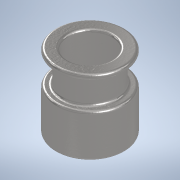
# Autodesk Inventor part: Umlenkrolle
Saved by Autodesk Inventor 2021 (Build 250183000, 183)
## iProperties
Created: 2020-05-16
Part Number: Umlenkrolle
Material: Generisch
Document SubType Name: Modeling
Designer: kaebi
Density: 1 g/cm^3
Appearance: Galvanized
Description: Antriebswelle Zahnriemen (Bestand)
Stock Number: -
Author: kaebi
Autodesk Inventor part; units mm, degrees
ref_plane "YZ Plane" through (0, 0, 0) normal (1, 0, 0) x (0, 1, 0)
ref_plane "XZ Plane" through (0, 0, 0) normal (0, 1, 0) x (-1, 0, 0)
ref_plane "XY Plane" through (0, 0, 0) normal (0, 0, 1) x (1, 0, 0)
sketch "Skizze1" plane through (0, 0, 0) normal (0, 0, 1) x (1, 0, 0)
  line L0 (0, 14) -> (-6.5, 14)
  line L1 (-6.5, 14) -> (-6.5, 13)
  line L2 (-6.5, 13) -> (-5, 13)
  line L3 (-5, 13) -> (-5, 8)
  line L4 (-5, 8) -> (-6.5, 8)
  line L5 (-6.5, 8) -> (-6.5, 0)
  line L6 (-6.5, 0) -> (0, 0)
  line L7 (0, 0) -> (-6.5, 0)
  line L8 (0, 0) -> (0, 14)
  line L9 (0, 13.1706) -> (0, 10.9789)
  dimension "d0" = 8
  dimension "d1" = 5
  dimension "d2" = 1
  dimension "d3" = 10
  dimension "d4" = 13
  constraints: 20 end point, 7 perpendicular, 2 collinear, 2 point on line, 1 horizontal
  measures "d0" distance of L4.end L5.end
  measures "d1" distance of L2.end L3.end
  measures "d2" distance of L0.end L1.end
  measures "d3" diameter of L3 L9
  measures "d4" diameter of L5 L9
revolve "Umdrehung1" add sketch "Skizze1" angle 360 about axis through (0, 13.1706, 0) along (0, -1, 0)
sketch "Sketch2" plane through (0, 14, 0) normal (0, 1, 0) x (1, 0, 0)
  circle A0 centre (0, 0) radius 4
  dimension "d6" = 8
  constraints: 1 centre point, 1 coincident
  measures "d6" diameter of A0
extrude "Extrusion1" cut sketch "Sketch2" against normal blind 20
fillet "Fillet1" radius 0.5 8 edges at (6.5, 14, 0) (6.5, 13, 0) (5, 8, 0) (6.5, 8, 0) (6.5, 0, 0) (5, 13, 0) (-4, 0, 0) (-4, 14, 0)
